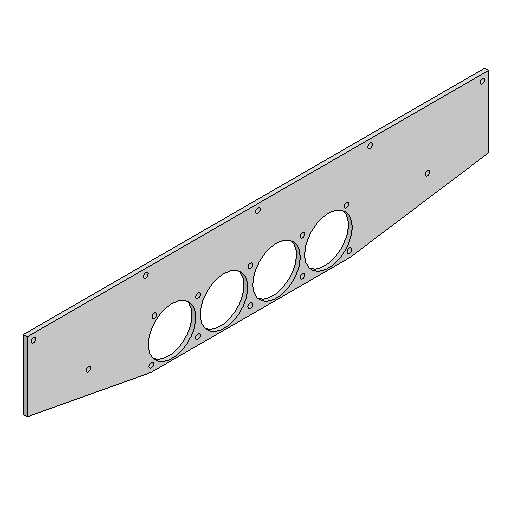
# Autodesk Inventor part: ChassiInsidePlate3.3
Saved by Autodesk Inventor 2023 (Build 270158000, 158)
## iProperties
Created: 2022-11-07
Part Number: ChassiInsidePlate3.3
Material: Generic
Document SubType Name: Modeling
Designer: deli
Density: 1 g/cm^3
Appearance: Default
Author: deli
Autodesk Inventor part; units mm, degrees
ref_plane "YZ Plane" through (0, 0, 0) normal (1, 0, 0) x (0, 1, 0)
ref_plane "XZ Plane" through (0, 0, 0) normal (0, 1, 0) x (-1, 0, 0)
ref_plane "XY Plane" through (0, 0, 0) normal (0, 0, 1) x (1, 0, 0)
sketch "Sketch1" plane through (0, 0, 0) normal (1, 0, 0) x (0, 1, 0)
  arc A0 (527.2088, -141.8041) -> (526.1602, -139.1772) centre (525.3711, -141.015) ccw projected
  arc A1 (236.0959, -13.3021) -> (237.3067, -15.1399) centre (238.0959, -13.3021) ccw projected
  line L0 (218.0959, 4.6452) -> (218.0959, 222.9071) projected
  line L1 (218.0959, 222.9071) -> (133.2497, 222.9071) projected
  line L2 (133.2497, 222.9071) -> (114.1833, 122.2834) projected
  arc A2 (114.1833, 122.2834) -> (114.0959, 121.3526) centre (119.0959, 121.3526) ccw projected
  arc A3 (114.0959, -41.0238) -> (114.1539, -41.7834) centre (119.0959, -41.0238) ccw projected
  line L3 (114.1539, -41.7834) -> (131.5694, -155.0929) projected
  line L4 (131.5694, -155.0929) -> (216.4156, -155.0929) projected
  circle A4 centre (185.0959, -150.0929) radius 2 projected
  circle A5 centre (185.0959, 125.9071) radius 2 projected
  circle A6 centre (153.0149, 118.7567) radius 2 projected
  circle A7 centre (152.8047, -38.6875) radius 2 projected
  circle A8 centre (142.0959, 172.9071) radius 2 projected
  circle A9 centre (142.0959, -105.0929) radius 2 projected
  circle A10 centre (134.8459, 104.2499) radius 4 projected
  circle A11 centre (134.8459, -23.9212) radius 4 projected
  circle A12 centre (149.3262, -2.6284) radius 2 projected
  circle A13 centre (120.3655, -2.6284) radius 2 projected
  circle A14 centre (185.0959, 217.9071) radius 2 projected
  circle A15 centre (185.0959, -58.0929) radius 2 projected
  circle A16 centre (185.0959, 33.9071) radius 2 projected
  circle A17 centre (119.0959, 121.3526) radius 2 projected
  circle A18 centre (119.0959, -41.0238) radius 2 projected
  line L5 (190.0959, 222.9071) -> (190.0959, -155.0929)
  circle A19 centre (134.8459, 104.2499) radius 19.5
  circle A20 centre (134.8459, -23.9212) radius 19.5
  line L6 (526.1602, -139.1772) -> (507.5647, -131.1921) projected
  line L7 (114.0959, 121.3526) -> (114.0959, -41.0238) projected
  line L8 (216.4156, -155.0929) -> (525.236, -146.3984) projected
  line L9 (525.236, -146.3984) -> (527.2088, -141.8041) projected
  circle A21 centre (257.849, -27.77) radius 1 projected
  circle A22 centre (340.5468, -63.2815) radius 1 projected
  circle A23 centre (437.0276, -104.7116) radius 1 projected
  circle A24 centre (519.7255, -140.2231) radius 1 projected
  arc A25 (505.0678, -124.9368) -> (507.5647, -131.1921) centre (509.4439, -126.816) ccw projected
  line L10 (505.0678, -124.9368) -> (507.7005, -118.8058) projected
  arc A26 (507.7005, -118.8058) -> (502.1873, -116.4383) centre (504.9439, -117.6221) ccw projected
  line L11 (502.1873, -116.4383) -> (499.5546, -122.5694) projected
  arc A27 (493.2993, -125.0664) -> (499.5546, -122.5694) centre (495.1785, -120.6903) ccw projected
  line L12 (493.2993, -125.0664) -> (237.3067, -15.1399) projected
  circle A28 centre (504.9439, -117.6221) radius 1.5 projected
  circle A29 centre (200.5959, 168.5571) radius 1.6 projected
  circle A30 centre (215.5959, 158.5571) radius 1.6 projected
  circle A31 centre (215.5959, 187.4571) radius 1.6 projected
  circle A32 centre (200.5959, 197.4571) radius 1.6 projected
  circle A33 centre (215.5959, 197.4571) radius 1.6 projected
  circle A34 centre (200.5959, 187.4571) radius 1.6 projected
  circle A35 centre (215.5959, 168.5571) radius 1.6 projected
  circle A36 centre (200.5959, 158.5571) radius 1.6 projected
  circle A37 centre (120.3655, 82.9571) radius 2 projected
  circle A38 centre (120.675, 40.1644) radius 2 projected
  circle A39 centre (134.8459, 18.6644) radius 4 projected
  circle A40 centre (134.8459, 61.6644) radius 4 projected
  circle A41 centre (149.0167, 40.1644) radius 2 projected
  circle A42 centre (149.3262, 82.9571) radius 2 projected
  circle A43 centre (134.8459, 61.6644) radius 19.5
  circle A44 centre (134.8459, 18.6644) radius 19.5
  line L13 (236.0959, -13.3021) -> (236.0959, -0.3548) projected
  arc A45 (236.0959, -0.3548) -> (233.0959, 2.6452) centre (233.0959, -0.3548) ccw projected
  line L14 (233.0959, 2.6452) -> (220.0959, 2.6452) projected
  arc A46 (218.0959, 4.6452) -> (220.0959, 2.6452) centre (220.0959, 4.6452) ccw projected
  circle A47 centre (233.0959, -0.3548) radius 2 projected
  point P0 (0, 0)
  point P1 (114.0959, 111.4062)
  dimension "d0" = 5
  dimension "d1" = 39
  constraints: 4 centre point, 4 coincident, 3 equal radius, 2 end point, 2 point on line, 1 vertical
  measures "d0" distance from line of L5 A5.centre
  measures "d1" diameter of A19
extrude "Extrusion1" add sketch "Sketch1" along normal blind 3.175 contours L4 L3 A3 L7 A2 L2 L1 L5
body "Solid1"
